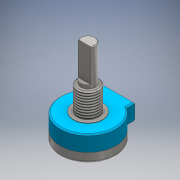
# Autodesk Inventor part: potenciometro
Saved by Autodesk Inventor 2016 (Build 200138000, 138)
## iProperties
Created: 2016-09-20
Part Number: potenciometro
Material: Acero inoxidable
Document SubType Name: Modeling
Designer: i95sa
Density: 8 g/cm^3
Appearance: Semipulido
Author: i95sa
Autodesk Inventor part; units mm, degrees
ref_plane "YZ Plane" through (0, 0, 0) normal (1, 0, 0) x (0, 1, 0)
ref_plane "XZ Plane" through (0, 0, 0) normal (0, 1, 0) x (-1, 0, 0)
ref_plane "XY Plane" through (0, 0, 0) normal (0, 0, 1) x (1, 0, 0)
sketch "Boceto1" plane through (0, 0, 0) normal (0, 0, 1) x (1, 0, 0)
  circle A0 centre (0, 0) radius 11.5
  dimension "d0" = 23
  constraints: 1 centre point, 1 coincident
  measures "d0" diameter of A0
extrude "Extrusión1" add sketch "Boceto1" along normal blind 4
sketch "Boceto2" plane through (0, 0, 4) normal (0, 0, 1) x (1, 0, 0)
  circle A0 centre (0, 0) radius 11.495
  dimension "d3" = 22.99
  constraints: 1 centre point, 1 coincident
  measures "d3" diameter of A0
extrude "Extrusión2" add sketch "Boceto2" along normal blind 0.01
sketch "Boceto3" plane through (0, 0, 4.01) normal (0, 0, 1) x (1, 0, 0)
  circle A0 centre (0, 0) radius 11.5
  line L0 (0, 0) -> (0, 11.5)
  line L1 (0, 13.1) -> (-6.25, 13.1)
  line L2 (-6.25, 13.1) -> (-6.25, 9.6534)
  line L3 (0, 13.1) -> (6.25, 13.1)
  line L4 (6.25, 13.1) -> (6.25, 9.6534)
  dimension "d6" = 23
  dimension "d22" = 13.1
  dimension "d23" = 6.25
  dimension "d24" = 6.25
  constraints: 10 end point, 3 point on circle, 2 horizontal, 2 perpendicular, 1 centre point, 1 coincident, 1 vertical
  measures "d6" diameter of A0
  measures "d22" distance of L0.start L1.start
  measures "d23" distance of L1.start L1.end
  measures "d24" distance of L1.start L3.end
extrude "Extrusión3" add sketch "Boceto3" along normal blind 6.52
sketch "Boceto4" plane through (0, 0, 10.53) normal (0, 0, 1) x (1, 0, 0)
  circle A0 centre (0, 0) radius 6
  dimension "d9" = 12
  constraints: 1 centre point, 1 coincident
  measures "d9" diameter of A0
extrude "Extrusión4" add sketch "Boceto4" along normal blind 0.2
sketch "Boceto5" plane through (0, 0, 10.73) normal (0, 0, 1) x (1, 0, 0)
  circle A0 centre (0, 0) radius 4.385
  dimension "d12" = 8.77
  constraints: 1 centre point, 1 coincident
  measures "d12" diameter of A0
extrude "Extrusión5" add sketch "Boceto5" along normal blind 10
sketch "Boceto6" plane through (0, 0, 20.73) normal (0, 0, 1) x (1, 0, 0)
  circle A0 centre (0, 0) radius 3
  dimension "d15" = 6
  constraints: 1 centre point, 1 coincident
  measures "d15" diameter of A0
extrude "Extrusión6" add sketch "Boceto6" along normal blind 1.5
sketch "Boceto7" plane through (0, 0, 22.23) normal (0, 0, 1) x (1, 0, 0)
  arc A0 (2.6263, -1.45) -> (-2.6263, -1.45) centre (0, 0) ccw
  circle A1 centre (0, 0) radius 3 projected
  line L0 (0, 0) -> (0, -1.45)
  line L1 (0, -1.45) -> (2.6263, -1.45)
  line L2 (0, -1.45) -> (-2.6263, -1.45)
  dimension "d19" = 1.45
  constraints: 6 end point, 4 point on circle, 1 centre point, 1 coincident, 1 horizontal, 1 perpendicular, 1 vertical
  measures "d19" distance of L0.start L0.end
extrude "Extrusión7" add sketch "Boceto7" along normal blind 13.56 contours L1 L2 A0
thread "Rosca1" size "M6x1" class "6g" standard "ANSI Metric M Profile" full length
fillet "Empalme1" radius 1 1 edges at (-11.5, 0, 0)
chamfer "Chaflán1" distance 0.5 angle 45 5 edges at (0, 13.1, 4.01) (0, 13.1, 10.53) (0, -11.5, 10.53) (-6.25, 11.3767, 10.53) (6.25, 11.3767, 10.53)
chamfer "Chaflán2" distance 0.3 angle 45 1 edges at (0, 3, 35.79)
chamfer "Chaflán3" distance 0.5 angle 45 1 edges at (-4.385, 0, 20.73)
